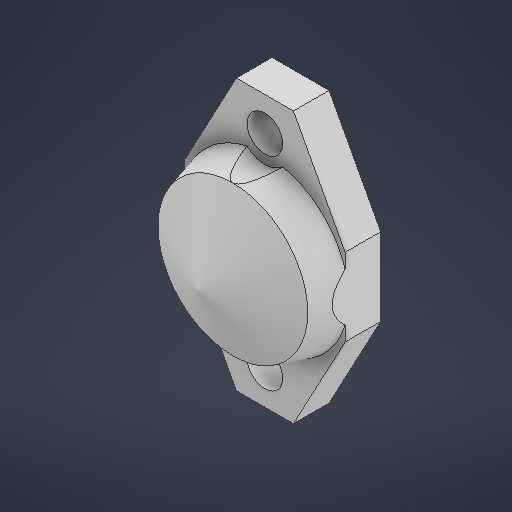
# Autodesk Inventor part: b10
Saved by Autodesk Inventor 2025.4 (Build 294407000, 407)
## iProperties
Created: 2026-05-15
Part Number: b10
Material: Generic
Document SubType Name: Modeling
Designer: VuQuan
Density: 1 g/cm^3
Appearance: Default
Author: VuQuan
Autodesk Inventor part; units mm, degrees
ref_plane "YZ Plane" through (0, 0, 0) normal (1, 0, 0) x (0, 1, 0)
sketch "Sketch1" plane through (0, 0, 0) normal (0, 0, 1) x (1, 0, 0)
  line L0 (-4.5, 0) -> (4.5, 0) construction
  line L1 (0, 7.6) -> (0, -7.6) construction
  line L2 (0, 7.6) -> (-1.6, 7.6)
  line L3 (-1.6, 7.6) -> (-4.5, 2.1794)
  line L4 (-4.5, 2.1794) -> (-4.5, 0)
  arc A0 (0, 5) -> (-4.5, 2.1794) centre (0, 0) ccw construction
  line L5 (0, 7.6) -> (1.6, 7.6)
  line L6 (1.6, 7.6) -> (4.5, 2.1794)
  line L7 (4.5, 2.1794) -> (4.5, 0)
  line L8 (0, -7.6) -> (-1.6, -7.6)
  line L9 (-1.6, -7.6) -> (-4.5, -2.1794)
  line L10 (-4.5, -2.1794) -> (-4.5, 0)
  line L11 (0, -7.6) -> (1.6, -7.6)
  line L12 (1.6, -7.6) -> (4.5, -2.1794)
  line L13 (4.5, -2.1794) -> (4.5, 0)
  point P0 (0, -5)
  dimension "d0" = 3.2
  dimension "d1" = 15.2
  dimension "d2" = 9
  dimension "d3" = 10
  constraints: 28 end point, 9 symmetric about line, 5 point on line, 2 coincident, 2 horizontal, 2 midpoint, 2 point on circle, 1 centre point, 1 vertical
  measures "d0" diameter of L2.end L1
  measures "d1" diameter of L2 L0
  measures "d2" diameter of L4 L1
  measures "d3" diameter of A0
extrude "Extrusion1" add sketch "Sketch1" along normal blind 2
sketch "Sketch2" plane through (0, 0, 0) normal (0, 0, 1) x (1, 0, 0)
  circle A0 centre (0, 5.7) radius 1
  circle A1 centre (0, -5.7) radius 1
  line L0 (-6.3, 0) -> (6.3, 0) projected
  point P0 (0, 0)
  dimension "d6" = 2
  dimension "d7" = 11.4
  constraints: 2 centre point, 2 vertical alignment, 1 equal radius, 1 symmetric about line
  measures "d6" diameter of A0
  measures "d7" distance of A1.centre A0.centre
extrude "Extrusion2" cut sketch "Sketch2" along normal through all
sketch "Sketch3" plane through (0, 0, 0) normal (1, 0, 0) x (0, 1, 0)
  line L0 (-6.7, 2) -> (-4.7, 2) projected
  line L1 (-4.7, 2) -> (-4.2, 3.8)
  line L2 (-4.2, 3.8) -> (0, 5.8)
  line L3 (0, 5.8) -> (4.2, 3.8) construction
  line L4 (4.7, 2) -> (6.7, 2) projected
  line L5 (4.2, 3.8) -> (4.7, 2) construction
  line L6 (0, 5.8) -> (0, 2)
  line L7 (2.1794, 2) -> (-2.1794, 2) projected
  line L8 (0, 2) -> (-4.7, 2)
  point P0 (0, 0)
  dimension "d10" = 5.8
  dimension "d11" = 3.8
  dimension "d12" = 8.4
  constraints: 12 end point, 2 equal length, 1 collinear, 1 horizontal alignment, 1 midpoint, 1 vertical alignment
  measures "d10" distance of point (0, 0) L2.end
  measures "d11" vertical distance of point (0, 0) L1.end
  measures "d12" distance of L3.end L1.end
revolve "Revolution1" add sketch "Sketch3" angle 360 about axis through (0, 0, 5.8) along (0, 0, -1)
sketch "Sketch4" plane through (0, 0, 2) normal (0, 0, 1) x (1, 0, 0)
  circle A0 centre (0, -5.7) radius 1 projected
  circle A1 centre (0, -5.7) radius 1.5
  circle A2 centre (0, 5.7) radius 1 projected
  circle A3 centre (0, 5.7) radius 1.5
  point P0 (0, 4.7)
  dimension "d14" = 3
  constraints: 2 centre point, 2 coincident, 1 equal radius, 1 vertical alignment
  measures "d14" diameter of A1
extrude "Extrusion3" cut sketch "Sketch4" along normal through all contours A0 | A1 | A2 | A3
sketch "Sketch5" plane through (0, 0, 0) normal (0, 0, -1) x (-1, 0, 0)
  circle A0 centre (0, 0) radius 3.5
  circle A1 centre (0, 0) radius 2.7
  dimension "d17" = 7
  dimension "d18" = 5.4
  constraints: 2 centre point, 2 coincident
  measures "d17" diameter of A0
  measures "d18" diameter of A1
extrude "Extrusion4" add sketch "Sketch5" along normal blind 0.8
ref_plane "Work Plane1" through (-4.5, -2.1794, 0) normal (-1, 0, 0) x (0, 0, 1)
split "Split1" plane through (-4.5, -2.1794, 0) removes the side toward (-1, 0, 0)
ref_plane "Work Plane2" through (4.5, -2.1794, 0) normal (1, 0, 0) x (0, 0, -1)
split "Split2" plane through (4.5, -2.1794, 0) removes the side toward (1, 0, 0)
body "Solid1"
